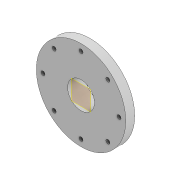
# Autodesk Inventor part: Cover of gearbox
Saved by Autodesk Inventor 2020.3 (Build 243373010, 373A)
## iProperties
Created: 2021-05-01
Part Number: Cover of gearbox
Material: Generic
Document SubType Name: Modeling
Designer: marti
Density: 1 g/cm^3
Appearance: Default
Author: marti
Autodesk Inventor part; units mm, degrees
ref_plane "YZ Plane" through (0, 0, 0) normal (1, 0, 0) x (0, 1, 0)
ref_plane "XZ Plane" through (0, 0, 0) normal (0, 1, 0) x (-1, 0, 0)
ref_plane "XY Plane" through (0, 0, 0) normal (0, 0, 1) x (1, 0, 0)
sketch "Sketch1" plane through (0, 0, 0) normal (0, 0, 1) x (1, 0, 0)
  circle A0 centre (0, 0) radius 50
  circle A1 centre (0, 0) radius 47.5
  circle A2 centre (0, 0) radius 42.5
  circle A3 centre (0, 0) radius 42.5
  circle A4 centre (0, 0) radius 42.5
  circle A5 centre (0, 0) radius 42.5
  circle A6 centre (0, 0) radius 42.5
  circle A7 centre (0, 0) radius 42.5
  circle A8 centre (0, 0) radius 42.5
  circle A9 centre (0, 0) radius 42.5
  point P0 (-42.5, 0)
  point P1 (-30.052, 30.052)
  point P2 (0, 42.5)
  point P3 (30.052, 30.052)
  point P4 (42.5, 0)
  point P5 (30.052, -30.052)
  point P6 (0, -42.5)
  point P7 (-30.052, -30.052)
  dimension "d4" = 85
  dimension "d0" = 100
  dimension "d3" = 95
  dimension "d5" = 360
  constraints: 2 centre point, 2 coincident, 2 horizontal alignment, 2 vertical alignment, 45 other
  measures "d0" diameter of A0
  measures "d3" diameter of A1
extrude "Extrusion1" add sketch "Sketch1" along normal blind 10 contours A0 | A1 | A2
hole "Hole1" at (-42.5, 0, 0) at (-30.052, 30.052, 0) at (0, 42.5, 0) at (30.052, 30.052, 0) at (42.5, 0, 0) at (30.052, -30.052, 0) at (0, -42.5, 0) at (-30.052, -30.052, 0) direction (0, 0, 1) diameter 4.4587 depth 10 tip angle 118 counterbore diameter 6 counterbore depth 2 thread size "M5x0.5" class "6H" standard "ISO Metric profile"
sketch "Sketch2" plane through (0, 0, 10) normal (0, 0, 1) x (1, 0, 0)
  circle A0 centre (0, 0) radius 21
  circle A1 centre (0, 0) radius 15
  dimension "d15" = 42
  dimension "d16" = 30
  constraints: 2 centre point, 2 coincident
  measures "d15" diameter of A0
  measures "d16" diameter of A1
ref_plane "Work Plane1" through (0, 0, 10) normal (0, 0, 1) x (1, 0, 0)
sketch "Sketch4" plane through (0, 0, 10) normal (0, 0, 1) x (1, 0, 0)
  circle A0 centre (0, 0) radius 15 projected
extrude "Extrusion4" cut sketch "Sketch4" against normal through all
sketch "Sketch5" plane through (0, 0, 0) normal (0, 0, -1) x (-1, 0, 0)
  circle A0 centre (0, 0) radius 32.5
  circle A1 centre (0, 0) radius 15 projected
  point P0 (0, 25)
  dimension "d23" = 25
  dimension "d24" = 65
  constraints: 1 centre point, 1 coincident
  measures "d23" distance of point (0, 0) point (0, 25)
  measures "d24" diameter of A0
extrude "Extrusion5" add sketch "Sketch5" along normal blind 10
body "Solid1"
